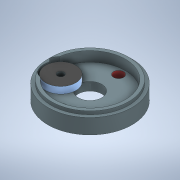
# Autodesk Inventor part: GEAR_BOTTOM
Saved by Autodesk Inventor 2020 (Build 240168000, 168)
## iProperties
Created: 2019-10-21
Part Number: GEAR_BOTTOM
Material: Ołów
Document SubType Name: Modeling
Designer: atmat
Density: 11.34 g/cm^3
Appearance: Ołów
Mass: 17.4719 g
Surface Area: 16.7882 cm^2
Volume: 1.54073 cm^3
Author: atmat
Autodesk Inventor part; units mm, degrees
ref_plane "YZ Plane" through (0, 0, 0) normal (1, 0, 0) x (0, 1, 0)
ref_plane "XZ Plane" through (0, 0, 0) normal (0, 1, 0) x (-1, 0, 0)
ref_plane "XY Plane" through (0, 0, 0) normal (0, 0, 1) x (1, 0, 0)
sketch "Szkic1" plane through (0, 0, 0) normal (0, 1, 0) x (-1, 0, 0)
  circle A0 centre (0, 0) radius 12.5
  dimension "d0" = 25
  constraints: 1 centre point, 1 coincident
  measures "d0" diameter of A0
extrude "Wyciągnięcie proste1" add sketch "Szkic1" along normal blind 2.5
sketch "Szkic2" plane through (0, 2.5, 0) normal (0, 1, 0) x (1, 0, 0)
  circle A0 centre (0, 0) radius 3.5
  dimension "d3" = 7
  constraints: 1 centre point, 1 coincident
  measures "d3" diameter of A0
extrude "Wyciągnięcie proste2" cut sketch "Szkic2" against normal blind 2.5
sketch "Szkic3" plane through (0, 2.5, 0) normal (0, 1, 0) x (1, 0, 0)
  circle A0 centre (0, -8.5) radius 1.5
  circle A1 centre (0, 8.5) radius 1.5
  point P0 (0, 0)
  dimension "d6" = 3
  dimension "d7" = 3
  dimension "d8" = 17
  dimension "d9" = 8.5
  constraints: 2 centre point
  measures "d6" diameter of A0
  measures "d7" diameter of A1
  measures "d8" distance of A1.centre A0.centre
  measures "d9" distance of A0.centre point (0, 0)
extrude "Wyciągnięcie proste3" cut sketch "Szkic3" against normal blind 2.5
sketch "Szkic4" plane through (0, 2.5, 0) normal (0, 1, 0) x (1, 0, 0)
  circle A0 centre (-6.7082, -2) radius 1
  circle A1 centre (-5.7446, 4) radius 1 construction
  point P0 (0, 0)
  dimension "d12" = 2
  dimension "d13" = 7
  dimension "d31" = 2
  dimension "d32" = 7
  dimension "d33" = 6
  dimension "d34" = 2
  constraints: 2 centre point
  measures "d12" diameter of A0
  measures "d13" distance of A0.centre point (0, 0)
  measures "d31" diameter of A1
  measures "d32" distance of point (0, 0) A1.centre
  measures "d33" vertical distance of A1.centre A0.centre
  measures "d34" vertical distance of point (0, 0) A0.centre
extrude "Wyciągnięcie proste4" cut sketch "Szkic4" against normal blind 2.5
sketch "Szkic6" plane through (0, 2.5, 0) normal (0, 1, 0) x (1, 0, 0)
  circle A0 centre (0, 0) radius 12.5
  circle A1 centre (0, 0) radius 10.5
  circle A2 centre (0, 0) radius 12.5 projected
  dimension "d19" = 2
  dimension "d20" = 0
  constraints: 2 centre point, 2 coincident
  measures "d19" radial gap between concentric circles of A1 A0
  measures "d20" radial gap between concentric circles of A2 A0
extrude "Wyciągnięcie proste6" add sketch "Szkic6" along normal blind 3
sketch "Szkic7" plane through (0, 5.5, 0) normal (0, 1, 0) x (1, 0, 0)
  circle A0 centre (0, 0) radius 12.5
  circle A1 centre (0, 0) radius 11.5
  circle A2 centre (0, 0) radius 12.5 projected
  dimension "d23" = 1
  dimension "d24" = 0
  constraints: 2 centre point, 2 coincident
  measures "d23" radial gap between concentric circles of A0 A1
  measures "d24" radial gap between concentric circles of A2 A0
extrude "Wyciągnięcie proste7" cut sketch "Szkic7" against normal blind 1
sketch "Szkic5" plane through (0, 2.5, 0) normal (0, 1, 0) x (1, 0, 0)
  circle A0 centre (-6.7082, -2) radius 5
  circle A1 centre (-6.7082, -2) radius 1 projected
  point P0 (0, 0)
  point P1 (-7, 0)
  dimension "d27" = 10
  constraints: 1 centre point, 1 concentric
  measures "d27" diameter of A0
extrude "Wyciągnięcie proste5" cut sketch "Szkic5" along normal blind 3 contours A0 | A1
sketch "Szkic8" plane through (0, 2.5, 0) normal (0, 1, 0) x (1, 0, 0)
  circle A0 centre (-6.7082, -2) radius 1 projected
  circle A1 centre (-6.7082, -2) radius 4.5
  point P0 (0, 0)
  dimension "d28" = 9
  constraints: 1 centre point, 1 coincident
  measures "d28" diameter of A1
extrude "Wyciągnięcie proste8" add sketch "Szkic8" along normal blind 2
sketch "Szkic9" plane through (0, 2.5, 0) normal (0, 1, 0) x (1, 0, 0)
  circle A0 centre (0, 0) radius 0.05
  dimension "d35" = 0.1
  constraints: 1 centre point, 1 coincident
  measures "d35" diameter of A0
extrude "Wyciągnięcie proste9" add sketch "Szkic9" along normal blind 2
